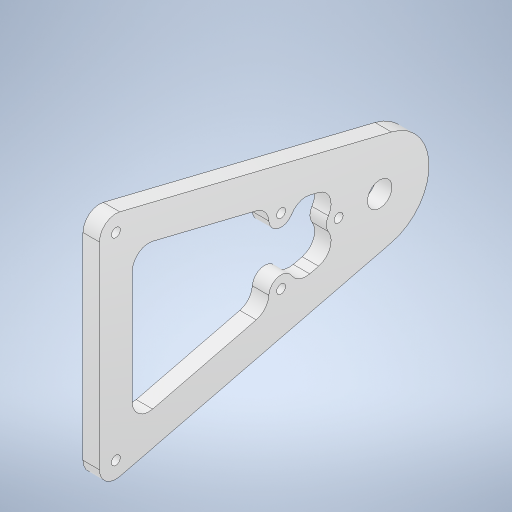
# Autodesk Inventor part: Upright - Blank
Saved by Autodesk Inventor 2023.4 (Build 274418000, 418)
## iProperties
Created: 2023-07-17
Part Number: Upright - Blank
Material: Aluminum 6061
Document SubType Name: Modeling
Designer: Nathan Cai
Mass: 56.1067 g
Surface Area: 124.558 cm^2
Volume: 20.7802 cm^3
Density: 2.7 g/cm^3
Appearance: Aluminum - Flat
Author: Nathan Cai
Autodesk Inventor part; units mm, degrees
ref_plane "YZ Plane" through (0, 0, 0) normal (1, 0, 0) x (0, 1, 0)
ref_plane "XZ Plane" through (0, 0, 0) normal (0, 1, 0) x (-1, 0, 0)
ref_plane "XY Plane" through (0, 0, 0) normal (0, 0, 1) x (1, 0, 0)
sketch "Sketch1" plane through (0, 0, 0) normal (1, 0, 0) x (0, 1, 0)
  circle A0 centre (0, 0) radius 3.5 construction
  circle A1 centre (38.1, -6.35) radius 1.7526
  circle A2 centre (38.1, -6.35) radius 6.35
  line L0 (0, 0) -> (0, -108.2802) construction
  circle A3 centre (0, -108.2802) radius 4.7625
  circle A4 centre (0, -108.2802) radius 19.05
  circle A5 centre (0, -92.4052) radius 1.7526
  circle A6 centre (0, -92.4052) radius 4.7625
  line L1 (44.2669, -7.8639) -> (18.5007, -112.8219)
  line L2 (31.9331, -4.8361) -> (10.4489, -92.3515)
  circle A7 centre (12.7, -70.1802) radius 1.7526
  circle A8 centre (12.7, -70.1802) radius 4.7625
  circle A9 centre (-38.1, -6.35) radius 1.7526
  circle A10 centre (-38.1, -6.35) radius 6.35
  line L3 (-44.2669, -7.8639) -> (-18.5007, -112.8219)
  line L4 (-31.9331, -4.8361) -> (-10.4489, -92.3515)
  circle A11 centre (-12.7, -70.1802) radius 1.7526
  circle A12 centre (-12.7, -70.1802) radius 4.7625
  line L5 (-38.1, 0) -> (38.1, 0)
  line L6 (38.1, -12.7) -> (-38.1, -12.7)
  point P0 (39.9083, -0.2629)
  point P1 (-39.9083, -0.2629)
  point P2 (-18.5007, -112.8219)
  point P3 (16.5723, -67.4078)
  point P4 (14.8483, -74.4306)
  point P5 (3.8683, -89.6271)
  point P6 (-3.8683, -89.6271)
  point P7 (-10.4489, -92.3515)
  point P8 (-14.8483, -74.4306)
  point P9 (-16.5723, -67.4078)
  point P10 (-30.0026, -12.7)
  point P11 (30.0026, -12.7)
  dimension "d0" = 7
  dimension "d2" = 3.5052
  dimension "d3" = 12.7
  dimension "d4" = 38.1
  dimension "d5" = 6.35
  dimension "d6" = 108.2802
  dimension "d7" = 9.525
  dimension "d8" = 38.1
  dimension "d9" = 3.5052
  dimension "d10" = 9.525
  dimension "d11" = 15.875
  dimension "d12" = 12.7
  dimension "d13" = 3.5052
  dimension "d14" = 9.525
  dimension "d15" = 12.7
  dimension "d16" = 38.1
  constraints: 14 end point, 13 centre point, 12 point on circle, 9 coincident, 9 symmetric about line, 6 tangent, 1 parallel, 1 point on line, 1 vertical, 4 other
  measures "d0" diameter of A0
  measures "d2" diameter of A1
  measures "d3" diameter of A2
  measures "d4" horizontal distance of L0.start A1.centre
  measures "d5" vertical distance of L0.start A1.centre
  measures "d6" distance of L0.start L0.end
  measures "d7" diameter of A3
  measures "d8" diameter of A4
  measures "d9" diameter of A5
  measures "d10" diameter of A6
  measures "d11" distance of A3.centre A6.centre
  measures "d12" distance between parallel lines of L1 L2
  measures "d13" diameter of A7
  measures "d14" diameter of A8
  measures "d15" distance from line of L0 A8.centre
  measures "d16" vertical distance of A3.centre A8.centre
extrude "Extrusion1" add sketch "Sketch1" along normal blind 6.35 contours A2 | A2 L2 L6 L4 A10 L5 | L1 A4 L2 A8 L6 A2 | A2 L6 L2 | A10 | A4 A6 | L4 L6 A10 | A10 L6 L4 A12 A4 L3 | A8 L2 | L2 A8 | A12 L4 | L4 A12 | A6 A4 | A4 A6
fillet "Fillet1" radius 6.35 10 edges at (3.175, 16.5723, -67.4078) (3.175, 14.8483, -74.4306) (3.175, 3.8683, -89.6271) (3.175, -3.8683, -89.6271) (3.175, -14.8483, -74.4306) (3.175, -16.5723, -67.4078) (3.175, 10.4489, -92.3515) (3.175, -10.4489, -92.3515) (3.175, -30.0026, -12.7) (3.175, 30.0026, -12.7)
equation "\"d4\" = S_Offset"
equation "\"d5\" = M2S"
equation "\"d6\" = C2C"
equation "\"d7\" = Bore"
equation "\"d8\" = FrontOD"
equation "\"d11\" = Leg_X_Front"
equation "\"d15\" = Leg_Y_Back"
equation "\"d16\" = Leg_X_Back"
equation "\"S_Offset\" = 38.1"
equation "\"M2S\" = 6.35"
equation "\"C2C\" = 108.2802"
equation "\"Bore\" = 9.525"
equation "\"FrontOD\" = 38.1"
equation "\"Leg_X_Front\" = 15.875"
equation "\"Leg_Y_Back\" = 12.7"
equation "\"Leg_X_Back\" = 38.1"
body "Solid1"
